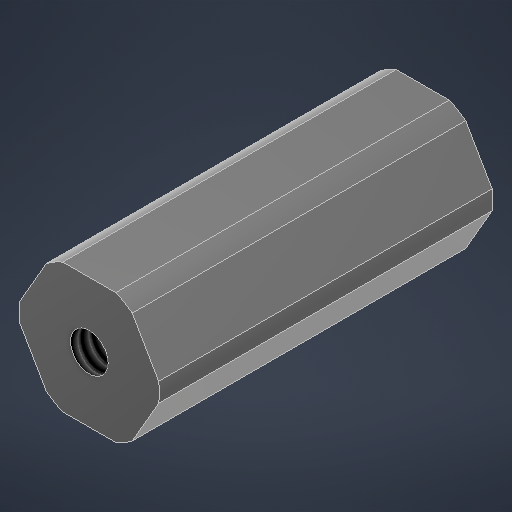
# Autodesk Inventor part: PINION_SHAFT_INTAKE
Saved by Autodesk Inventor 2026.2 (Build 302298010, 298A)
## iProperties
Created: 2026-04-02
Part Number: PINION_SHAFT_INTAKE
Material: Aluminum, 7075-T6
Document SubType Name: Modeling
Designer: 4aida
Density: 2.81 g/cm^3
Appearance: Smooth - Black
Author: 4aida
Autodesk Inventor part; units mm, degrees
ref_plane "YZ Plane" through (0, 0, 0) normal (1, 0, 0) x (0, 1, 0)
ref_plane "XZ Plane" through (0, 0, 0) normal (0, 1, 0) x (-1, 0, 0)
ref_plane "XY Plane" through (0, 0, 0) normal (0, 0, 1) x (1, 0, 0)
sketch "Sketch1" plane through (0, 0, 0) normal (0, 0, 1) x (1, 0, 0)
  line L0 (-3.6662, 6.35) -> (3.6662, 6.35)
  line L1 (3.6662, 6.35) -> (7.3323, 0)
  line L2 (7.3323, 0) -> (3.6662, -6.35)
  line L3 (3.6662, -6.35) -> (-3.6662, -6.35)
  line L4 (-3.6662, -6.35) -> (-7.3323, 0)
  line L5 (-7.3323, 0) -> (-3.6662, 6.35)
  circle A0 centre (0, 0) radius 6.858
  point P0 (2.5903, -6.35)
  point P1 (4.2041, -5.4183)
  point P2 (6.7944, -0.9317)
  point P3 (6.7944, 0.9317)
  point P4 (4.2041, 5.4183)
  point P5 (2.5903, 6.35)
  point P6 (-2.5903, 6.35)
  point P7 (-4.2041, 5.4183)
  point P8 (-6.7944, 0.9317)
  point P9 (-6.7944, -0.9317)
  point P10 (-4.2041, -5.4183)
  point P11 (-2.5903, -6.35)
  dimension "d0" = 12.7
  dimension "d1" = 13.716
  constraints: 12 end point, 2 coincident, 1 centre point, 1 horizontal, 13 other
  measures "d0" distance between parallel lines of L3 L0
  measures "d1" diameter of A0
extrude "Extrusion1" add sketch "Sketch1" along normal mid plane 32.639 contours L0 A0 L1 L2 L3 L4 L5
sketch "Sketch2" plane through (0, 0, 16.3195) normal (0, 0, 1) x (1, 0, 0)
  point P0 (0, 0)
hole "Hole1" at (0, 0, 16.3195) direction (0, 0, -1) diameter 3.683 end through all thread size "10-24 UNC" class "2B" standard "ANSI Unified Screw Threads"
mirror "Mirror1" about plane through (0, 0, 0) normal (0, 0, 1) of "Hole1"
body "Solid1"
